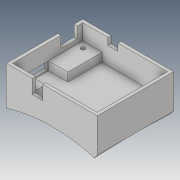
# Autodesk Inventor part: Base
Saved by Autodesk Inventor 2017 (Build 210142000, 142)
## iProperties
Created: 2017-03-19
Part Number: Base
Material: Generic
Document SubType Name: Modeling
Designer: Liam
Density: 1 g/cm^3
Appearance: Default
Author: Liam
Autodesk Inventor part; units mm, degrees
ref_plane "YZ Plane" through (0, 0, 0) normal (1, 0, 0) x (0, 1, 0)
ref_plane "XZ Plane" through (0, 0, 0) normal (0, 1, 0) x (-1, 0, 0)
sketch "Sketch1" plane through (0, 0, 0) normal (0, 1, 0) x (-1, 0, 0)
  line L0 (0, 0) -> (67.9, 0)
  line L1 (67.9, 0) -> (67.9, -56.3)
  line L2 (67.9, -56.3) -> (0, -56.3)
  line L3 (0, -56.3) -> (0, 0)
  dimension "d4" = 67.9
  dimension "d5" = 56.3
  constraints: 8 end point, 2 parallel, 1 horizontal, 1 perpendicular
  measures "d4" distance of L0.start L0.end
  measures "d5" distance of L0.end L1.end
extrude "Extrusion1" add sketch "Sketch1" along normal blind 2
sketch "Sketch4" plane through (0, 0, 0) normal (0, -1, 0) x (1, 0, 0)
  line L0 (2.5, 2.5) -> (-70.4, 2.5)
  line L1 (-70.4, 2.5) -> (-70.4, -58.8)
  line L2 (-70.4, -58.8) -> (2.5, -58.8)
  line L3 (2.5, -58.8) -> (2.5, 2.5)
  line L4 (0, -56.3) -> (0, 0) projected
  line L5 (0, 0) -> (-67.9, 0) projected
  line L6 (-67.9, -56.3) -> (0, -56.3) projected
  line L7 (-67.9, -56.3) -> (-67.9, 0) projected
  line L8 (0, 0) -> (-67.9, 0)
  line L9 (-67.9, 0) -> (-67.9, -56.3)
  line L10 (-67.9, -56.3) -> (0, -56.3)
  line L11 (0, -56.3) -> (0, 0)
  point P0 (-67.7799, -40.4535)
  point P1 (-67.7799, -17.6706)
  dimension "d35" = 2.5
  dimension "d36" = 2.5
  dimension "d37" = 2.5
  dimension "d38" = 2.5
  constraints: 16 end point, 4 parallel, 2 horizontal, 2 perpendicular, 1 other
  measures "d35" distance between parallel lines of L4 L3
  measures "d36" distance between parallel lines of L5 L0
  measures "d37" distance between parallel lines of L6 L2
extrude "Extrusion3" add sketch "Sketch4" against normal blind 21.7
sketch "Sketch5" plane through (2.5, 0, -58.8) normal (0, 0, -1) x (-1, 0, 0)
  line L0 (0, 0) -> (0, -5.5)
  line L1 (0, 0) -> (35.56, 0)
  line L2 (0, 0) -> (72.9, 0) projected
  arc A0 (35.56, 0) -> (0, -5.5) centre (35.56, -117.7058) ccw
  line L3 (72.9, 0) -> (0, 0) projected
  point P0 (2.5, 0)
  dimension "d41" = 5.5
  dimension "d42" = 35.56
  constraints: 4 end point, 2 point on circle, 2 point on line, 1 centre point, 1 tangent, 1 vertical
  measures "d41" distance of L0.start L0.end
  measures "d42" distance of L1.end L0.start
extrude "Extrusion4" add sketch "Sketch5" against normal up to surface (61.3 mm away)
ref_plane "Work Plane1" through (-33.95, 21.7, 2.5) normal (1, 0, 0) x (0, 0, -1)
mirror "Mirror1" about plane through (-33.95, 21.7, 2.5) normal (1, 0, 0) of "Extrusion4"
sketch "Sketch11" plane through (0, 2, 0) normal (0, 1, 0) x (1, 0, 0)
  line L0 (-67.9, 0) -> (0, 0) projected
  line L1 (0, 0) -> (0, 56.3) projected
  line L2 (0, 56.3) -> (-67.9, 56.3) projected
  line L3 (-67.9, 56.3) -> (-67.9, 0) projected
  line L4 (-67.9, 0) -> (-52.5, 0)
  line L5 (-52.5, 0) -> (-52.5, 10.9)
  line L6 (-52.5, 10.9) -> (-67.9, 10.9)
  line L7 (-67.9, 10.9) -> (-67.9, 0)
  line L8 (-67.9, 56.3) -> (-52.4, 56.3)
  line L9 (-52.4, 56.3) -> (-52.4, 28.9)
  line L10 (-52.4, 28.9) -> (-67.9, 28.9)
  line L11 (-67.9, 28.9) -> (-67.9, 56.3)
  line L12 (0, 0) -> (-16.2, 0)
  line L13 (-16.2, 0) -> (-16.2, 12.4)
  line L14 (-16.2, 12.4) -> (0, 12.4)
  line L15 (0, 12.4) -> (0, 0)
  line L16 (0, 0) -> (0, 56.3) projected
  line L17 (0, 56.3) -> (-4, 56.3)
  line L18 (-4, 56.3) -> (-4, 29)
  line L19 (-4, 29) -> (0, 29)
  line L20 (0, 29) -> (0, 56.3)
  dimension "d89" = 15.4
  dimension "d90" = 10.9
  dimension "d91" = 15.5
  dimension "d92" = 27.4
  dimension "d93" = 16.2
  dimension "d94" = 12.4
  dimension "d95" = 4
  dimension "d96" = 27.3
  constraints: 32 end point, 8 parallel, 4 horizontal, 4 perpendicular
  measures "d89" distance of L6.end L5.end
  measures "d90" distance of L5.end L4.end
  measures "d91" distance of L9.end L10.end
  measures "d92" distance of L8.end L9.end
  measures "d93" distance of L13.end L14.end
  measures "d94" distance of L12.end L13.end
  measures "d95" distance of L19.end L18.end
  measures "d96" distance of L18.end L17.end
extrude "Extrusion7" add sketch "Sketch11" along normal blind 7 contours L3 L6 L5 L0 | L13 L14 L1 L0 | L3 L2 L9 L10 | L19 L18 L2 L1
sketch "Sketch12" plane through (0, 9, 0) normal (0, 1, 0) x (1, 0, 0)
  line L0 (0, 0) -> (-67.9, 0) projected
  line L1 (-67.9, 0) -> (-67.9, 56.3) projected
  line L2 (-67.9, 56.3) -> (0, 56.3) projected
  line L3 (0, 56.3) -> (0, 0) projected
  point P0 (-62.6, 5.2)
  point P1 (-5.3, 5)
  point P2 (-62.7, 51.3)
  dimension "d99" = 5.2
  dimension "d100" = 5.3
  dimension "d101" = 5.2
  dimension "d102" = 5
  dimension "d103" = 5
  dimension "d104" = 5.3
  measures "d99" distance from line of L0 point (-62.6, 5.2)
  measures "d100" distance from line of point (-62.6, 5.2) L1
  measures "d101" distance from line of point (-62.7, 51.3) L1
  measures "d102" distance from line of point (-62.7, 51.3) L2
  measures "d103" distance from line of point (-5.3, 5) L0
  measures "d104" distance from line of L3 point (-5.3, 5)
hole "Hole6" at (-62.6, 9, -5.2) at (-5.3, 9, -5) at (-62.7, 9, -51.3) direction (0, -1, 0) diameter 3.3 depth 9
sketch "Sketch13" plane through (-70.4, 0, 2.5) normal (0, 0, 1) x (1, 0, 0)
  line L0 (17.9, 9) -> (2.5, 9) projected
  line L1 (70.4, 9) -> (54.2, 9) projected
  line L2 (20.8, 10.6) -> (29.4, 10.6)
  line L3 (29.4, 10.6) -> (29.4, 21.7)
  line L4 (29.4, 21.7) -> (20.8, 21.7)
  line L5 (20.8, 21.7) -> (20.8, 10.6)
  line L6 (0, 21.7) -> (72.9, 21.7) projected
  point P0 (70.4, 0)
  point P1 (2.5, 21.7)
  dimension "d112" = 1.6
  dimension "d113" = 18.3
  dimension "d114" = 8.6
  constraints: 8 end point, 2 parallel, 1 collinear, 1 horizontal, 1 perpendicular
  measures "d112" distance between parallel lines of L2 L0
  measures "d113" distance from line of L0.end L5
  measures "d114" distance of L3.end L4.end
extrude "Extrusion8" cut sketch "Sketch13" against normal up to surface (2.5 mm away)
sketch "Sketch14" plane through (-70.4, 0, -58.8) normal (-1, 0, 0) x (0, 0, 1)
  line L0 (5.85, 9) -> (9.15, 9) projected
  line L1 (29.9, 9) -> (2.5, 9) projected
  line L2 (29.9, 9) -> (2.5, 9) projected
  line L3 (58.8, 9) -> (47.9, 9) projected
  line L4 (51.95, 9) -> (55.25, 9) projected
  line L5 (58.8, 9) -> (47.9, 9) projected
  line L6 (58.8, 9) -> (47.9, 9) projected
  line L7 (30.4, 9) -> (47.4, 9)
  line L8 (47.4, 9) -> (47.4, 3)
  line L9 (47.4, 3) -> (30.4, 3)
  line L10 (30.4, 3) -> (30.4, 9)
  point P0 (58.8, 0)
  dimension "d118" = 11.4
  dimension "d119" = 17
  dimension "d120" = 6
  constraints: 8 end point, 2 parallel, 1 collinear, 1 horizontal, 1 perpendicular
  measures "d118" distance from line of L3.start L8
  measures "d119" distance of L7.start L7.end
  measures "d120" distance of L9.end L7.start
extrude "Extrusion9" cut sketch "Sketch14" against normal up to surface (2.5 mm away)
sketch "Sketch15" plane through (2.5, 0, -58.8) normal (0, 0, -1) x (-1, 0, 0)
  line L0 (63.55, 9) -> (66.85, 9) projected
  line L1 (70.4, 9) -> (54.9, 9) projected
  line L2 (70.4, 9) -> (54.9, 9) projected
  line L3 (6.5, 9) -> (2.5, 9) projected
  line L4 (6.5, 9) -> (2.5, 9) projected
  line L5 (50.2, 21.7) -> (50.2, 16)
  line L6 (50.2, 16) -> (42.2, 16)
  line L7 (42.2, 16) -> (42.2, 21.7)
  line L8 (37.34, 0) -> (35.56, 0) projected
  line L9 (72.9, 21.7) -> (72.9, -5.5) projected
  line L10 (0, 21.7) -> (72.9, 21.7) projected
  line L11 (0, 21.7) -> (0, -5.5) projected
  arc A0 (35.56, 0) -> (0, -5.5) centre (35.56, -117.7058) ccw projected
  arc A1 (72.9, -5.5) -> (37.34, 0) centre (37.34, -117.7058) ccw projected
  line L12 (54.9, 2) -> (70.4, 2) projected
  line L13 (70.4, 2) -> (55, 2) projected
  line L14 (55, 2) -> (18.7, 2) projected
  line L15 (18.7, 2) -> (2.5, 2) projected
  line L16 (2.5, 2) -> (6.5, 2) projected
  line L17 (6.5, 2) -> (54.9, 2) projected
  line L18 (6.15, 9) -> (9.45, 9) projected
  line L19 (2.5, 9) -> (18.7, 9) projected
  line L20 (2.5, 9) -> (18.7, 9) projected
  point P0 (2.5, 0)
  dimension "d124" = 39.7
  dimension "d126" = 7
  dimension "d127" = 8
  constraints: 6 end point, 2 point on line, 1 parallel, 1 vertical
  measures "d124" distance from line of L3.end L7
  measures "d126" distance between parallel lines of L1 L6
  measures "d127" distance of L5.end L6.end
extrude "Extrusion10" cut sketch "Sketch15" against normal up to surface (2.5 mm away) contours L5 L6 L7 L10
sketch "Sketch16" plane through (-70.4, 21.7, -58.8) normal (-1, 0, 0) x (0, 0, 1)
  line L0 (0, -21.7) -> (61.3, -21.7) projected
  line L1 (0, -27.2) -> (0, -21.7) projected
  line L2 (61.3, 0) -> (61.3, -27.2) projected
  line L3 (0, -27.2) -> (61.3, -27.2) projected
  arc A0 (61.3, -31.2) -> (0, -31.2) centre (30.65, -146.6278) ccw
  line L4 (0, -27.2) -> (61.3, -27.2) projected
  line L5 (0, -31.2) -> (0, -27.2)
  line L6 (61.3, -27.2) -> (61.3, -31.2)
  point P0 (58.8, -21.7)
  point P1 (30.65, -26.2)
  dimension "d134" = 4
  dimension "d136" = 4
  constraints: 4 end point, 2 point on circle, 1 centre point, 1 parallel, 1 tangent, 1 vertical
  measures "d134" distance from line of L5.start L3
  measures "d136" distance of L2.end L6.end
sketch3d "3D Sketch1"
  arc A0 (-70.4, -5.5, -58.8) -> (-34.84, 0, -58.8) centre (-34.84, -117.7058, -58.8) ccw
  line L0 (-34.84, 0, -58.8) -> (-33.06, 0, -58.8)
  arc A1 (-33.06, 0, -58.8) -> (2.5, -5.5, -58.8) centre (-33.06, -117.7058, -58.8) ccw
sweep "Sweep1" add profiles "Sketch16" path "3D Sketch1" contours L3 A0 L5 | L6 A0 L3
sketch "Sketch17" plane through (-70.4, 21.7, -58.8) normal (-1, 0, 0) x (0, 0, 1)
  line L0 (30.4, -12.7) -> (47.4, -12.7) projected
  line L1 (47.4, -12.7) -> (47.4, -18.7) projected
  line L2 (47.4, -18.7) -> (30.4, -18.7) projected
  line L3 (30.4, -18.7) -> (30.4, -12.7) projected
  line L4 (61.3, 0) -> (61.3, -31.2) projected
  line L5 (0, 0) -> (61.3, 0) projected
  line L6 (0, 0) -> (0, -31.2) projected
  arc A0 (61.3, -31.2) -> (0, -31.2) centre (30.65, -146.6278) ccw projected
  line L7 (2.5, 0) -> (58.8, 0) projected
  line L8 (7, 0) -> (20, 0)
  line L9 (20, 0) -> (20, -9)
  line L10 (20, -9) -> (7, -9)
  line L11 (7, -9) -> (7, 0)
  point P0 (58.8, -21.7)
  dimension "d139" = 13
  dimension "d140" = 9
  dimension "d141" = 7
  constraints: 8 end point, 2 parallel, 1 horizontal, 1 perpendicular, 1 point on line
  measures "d139" distance of L9.end L10.end
  measures "d140" distance of L8.end L9.end
  measures "d141" distance between parallel lines of L11 L6
extrude "Extrusion11" cut sketch "Sketch17" against normal up to surface (2.5 mm away) contours L9 L10 L11 L5
sketch "Sketch18" plane through (-67.9, 9, 0) normal (1, 0, 0) x (0, 0, -1)
  line L0 (51.8, 12.7) -> (51.8, 3.7) projected
  line L1 (51.8, 3.7) -> (38.8, 3.7) projected
  line L2 (38.8, 3.7) -> (38.8, 12.7) projected
  line L3 (0, 12.7) -> (38.8, 12.7) projected
  line L4 (0, 0) -> (0, 12.7) projected
  line L5 (0, 0) -> (10.9, 0) projected
  line L6 (10.9, 0) -> (10.9, -7) projected
  line L7 (28.9, -7) -> (10.9, -7) projected
  line L8 (28.9, -7) -> (28.9, 0) projected
  line L9 (28.9, 0) -> (56.3, 0) projected
  line L10 (56.3, 0) -> (56.3, 12.7) projected
  line L11 (51.8, 12.7) -> (56.3, 12.7) projected
  line L12 (11.4, 0) -> (28.4, 0) projected
  line L13 (28.4, 0) -> (28.4, -6) projected
  line L14 (28.4, -6) -> (11.4, -6) projected
  line L15 (11.4, -6) -> (11.4, 0) projected
  line L16 (10.9, 3.7) -> (45.4, 3.7)
  line L17 (45.4, 3.7) -> (45.4, 1.7)
  line L18 (45.4, 1.7) -> (10.9, 1.7)
  line L19 (10.9, 1.7) -> (10.9, 3.7)
  line L20 (51.8, 3.7) -> (38.8, 3.7) projected
  line L21 (10.9, 0) -> (10.9, -7) projected
  point P0 (0, -9)
  dimension "d145" = 1.7
  dimension "d147" = 10.9
  constraints: 8 end point, 2 collinear, 2 parallel, 1 horizontal, 1 perpendicular
  measures "d145" distance between parallel lines of L9 L18
  measures "d147" distance between parallel lines of L10 L17
body "Solid1"
